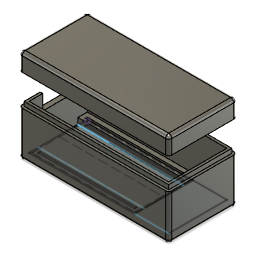
ReceiverCase (Autodesk Fusion 360 design; units mm, degrees)
Autodesk Fusion 360 part; units mm, degrees
note: some values were not read from the file. Set by a fixed rule: which face or edge a step refers to.
sketch "Sketch1" plane through (0, 0, 0) normal (0, 1, 0) x (1, 0, 0) in component "Case Bottom"
  line L0 (0, 0) -> (33.02, 0) construction
  line L1 (33.02, 0) -> (33.02, -17.78) construction
  line L2 (33.02, -17.78) -> (0, -17.78) construction
  line L3 (0, -17.78) -> (0, 0) construction
  line L4 (0, 0) -> (33.02, 0) construction
  line L5 (33.02, -2.54) -> (0, -2.54) construction
  line L6 (0, -2.54) -> (0, 0) construction
  line L7 (0, -17.78) -> (33.02, -17.78) construction
  line L8 (33.02, -17.78) -> (33.02, -15.24) construction
  line L9 (33.02, -15.24) -> (0, -15.24) construction
  line L10 (0, -15.24) -> (0, -17.78) construction
  line L11 (0, -8.89) -> (33.02, -8.89) construction
  line L12 (0.945, -0.945) -> (32.075, -0.945)
  line L13 (32.075, -0.945) -> (32.075, -1.595)
  line L14 (32.075, -1.595) -> (0.945, -1.595)
  line L15 (0.945, -1.595) -> (0.945, -0.945)
  line L16 (32.075, -16.835) -> (32.075, -16.185)
  line L17 (0.945, -16.185) -> (0.945, -16.835)
  line L18 (32.075, -16.185) -> (0.945, -16.185)
  line L19 (0.945, -16.835) -> (32.075, -16.835)
  line L20 (-0.5, -18.28) -> (-0.5, 0.5)
  line L21 (-0.5, 0.5) -> (33.52, 0.5)
  line L22 (33.52, 0.5) -> (33.52, -18.28)
  line L23 (33.52, -18.28) -> (-0.5, -18.28)
  line L24 (33.52, 0.5) -> (44.52, 0.5)
  line L25 (44.52, 0.5) -> (44.52, -18.28)
  line L26 (44.52, -18.28) -> (33.52, -18.28)
  line L27 (33.52, -18.28) -> (33.52, 0.5)
  line L28 (-0.5, -2.54) -> (33.52, -2.54)
  line L29 (33.52, -15.24) -> (-0.5, -15.24)
  dimension "d1" = 33.02
  dimension "d2" = 17.78
  dimension "d3" = 2.54
  dimension "d4" = 2.54
  dimension "d15" = 0.945
  dimension "d16" = 0.945
  dimension "d17" = 0.65
  dimension "d18" = 0.945
  dimension "d19" = -0.5
  dimension "d21" = 11
  constraint horizontal L0
  constraint vertical L1
  constraint horizontal L2
  constraint vertical L3
  constraint coincident L0.start L3.end
  constraint horizontal L4
  constraint horizontal L5
  constraint vertical L6
  constraint horizontal L7
  constraint vertical L8
  constraint coincident L1 L8.end
  constraint midpoint L3 L11.start
  constraint midpoint L1 L11.end
  constraint coincident L1 L5.start
  constraint horizontal L12
  constraint vertical L13
  constraint horizontal L14
  constraint vertical L15
  constraint symmetric L11 L12.start L17.end
  constraint symmetric L11 L12.end L16.start
  constraint symmetric L11 L13.end L16.end
  constraint symmetric L11 L14.end L17.start
  constraint horizontal L24
  constraint vertical L25
  constraint horizontal L26
  constraint vertical L27
  constraint coincident L20 L28.start
  constraint coincident L27 L28.end
  constraint perpendicular L27 L28
  constraint coincident L27 L29.start
  constraint coincident L20 L29.end
  constraint perpendicular L20 L29
  measures "d1" distance of L0.start L0.end
  measures "d2" distance of L0.start L2.end
  measures "d3" distance of L0.start L5.end
  measures "d4" distance of L2.end L9.end
  measures "d15" distance of L1 L13
  measures "d16" distance of L6 L15
  measures "d17" distance of L12 L14
  measures "d18" distance of L4 L12
  measures "d21" distance of L21.end L24.end
extrude "Extrude1" add sketch "Sketch1" along normal blind 17 contours L12 L13 L14 L15 | L16 L17 L18 L19 | L20 L22 L23 L27 L29 | L20 L22 L27 L28 L29 | L22 L24 L25 L26 L27 | L20 L21 L22 L27 L28 makes body 1 in component "Case Bottom"
shell "Shell1" thickness 1.6 outward yes removed faces 0 bodies 1 in component "Case Bottom"
ref_plane "WorkPlane2" through (22.01, 13, 8.89) normal (0, 1, 0) x (1, 0, 0) in component "Case Bottom"
split "Split2" by plane through (22.01, 13, 8.89) normal (0, 1, 0) bodies 1 makes body 2 at (13.9733, 18.6, 5.2267) in component "Case Bottom"
extrude "Extrude3" add sketch "Sketch1" along normal blind 2 contours L20 L22 L23 L27 L29 | L20 L21 L22 L27 L28 bodies 1 in component "Case Bottom"
sketch "Sketch2" plane through (-2.1, 0, 0) normal (-1, 0, 0) x (0, 0, 1) in component "Case Bottom"
  line L0 (19.88, 13) -> (-2.1, 13)
  line L1 (-2.1, 13) -> (-2.1, -1.6)
  line L2 (-2.1, -1.6) -> (19.88, -1.6)
  line L3 (19.88, -1.6) -> (19.88, 13)
  line L4 (18.28, 13) -> (-0.5, 13)
  line L5 (-0.5, 13) -> (-0.5, 0)
  line L6 (-0.5, 0) -> (18.28, 0)
  line L7 (18.28, 0) -> (18.28, 13)
  line L8 (8.89, 13) -> (8.89, 0) construction
  line L9 (3.89, 13) -> (13.89, 13)
  line L10 (13.89, 13) -> (13.89, 9.5)
  line L11 (13.89, 9.5) -> (3.89, 9.5)
  line L12 (3.89, 9.5) -> (3.89, 13)
  dimension "d30" = 9.5
  dimension "d31" = 5
  dimension "d32" = 5
  constraint midpoint L4 L8.start
  constraint midpoint L6 L8.end
  constraint horizontal L9
  constraint vertical L10
  constraint horizontal L11
  constraint vertical L12
  constraint coincident L4 L9.start
  measures "d30" distance of L6 L11
  measures "d31" distance of L8 L12
  measures "d32" distance of L8 L10
extrude "Extrude4" cut sketch "Sketch2" against normal up to surface (1.6 mm away) contours L0 L4 L9 L10 L11 L12 bodies 1 in component "Case Bottom"
fillet "Fillet1" radius 1 2 edges at (46.12, 5.7, 19.88) (46.12, 5.7, -2.1) on bodies 1 in component "Case Bottom"
fillet "Fillet2" radius 1 2 edges at (-2.1, 5.7, -2.1) (-2.1, 5.7, 19.88) on bodies 1 in component "Case Bottom"
ref_plane "WorkPlane3" through (22.01, 11.4, 8.89) normal (0, 1, 0) x (0, 0, 1) in component "Case Bottom"
split_face "SplitFace1" 4 faces at (25.8467, 9.3333, -0.5) (-0.5, 4.5, 10.5567) (25.8467, 9.3333, 18.28) (44.52, 4.3333, 5.76) by plane through (22.01, 11.4, 8.89) normal (0, 1, 0) on bodies 1 in component "Case Bottom"
move_face "OffsetFaces1" offset -0.8 5 faces at (14.5067, 11.9333, -0.5) (-0.5, 11.9333, 2.4267) (-0.5, 11.9333, 16.8167) (29.5133, 11.9333, 18.28) (44.52, 12.4667, 5.76) on bodies 1 in component "Case Bottom"
sketch "Sketch4" plane through (44.52, 0, 0) normal (-1, 0, 0) x (0, 0, 1) in component "Case Bottom"
  line L0 (18.28, 11.4) -> (-0.5, 11.4)
  line L1 (-0.5, 11.4) -> (-0.5, 0)
  line L2 (-0.5, 0) -> (18.28, 0)
  line L3 (18.28, 0) -> (18.28, 11.4)
  line L4 (4.755, 10) -> (13.025, 10)
  line L5 (13.025, 10) -> (13.025, 9.35)
  line L6 (13.025, 9.35) -> (4.755, 9.35)
  line L7 (4.755, 9.35) -> (4.755, 10)
  line L8 (8.89, 13) -> (8.89, 0) construction
  line L9 (-0.5, 0) -> (18.28, 0)
  line L10 (14.025, 8.35) -> (3.755, 8.35)
  line L11 (3.755, 8.35) -> (3.755, 11)
  line L12 (3.755, 11) -> (14.025, 11)
  line L13 (14.025, 11) -> (14.025, 8.35)
  dimension "d43" = 8.27
  dimension "d44" = 0.65
  dimension "d45" = 4.135
  dimension "d46" = 9.35
  dimension "d47" = -1
  constraint horizontal L4
  constraint vertical L5
  constraint horizontal L6
  constraint vertical L7
  measures "d43" distance of L4.start L4.end
  measures "d44" distance of L4.start L6.end
  measures "d45" distance of L7 L8
  measures "d46" distance of L6 L9
extrude "Extrude5" add sketch "Sketch4" along normal blind 1.6 contours L10 L11 L12 L13 bodies 1 in component "Case Bottom"
fillet "Fillet3" radius 1 4 edges at (-2.1, 15.8, 19.88) (-2.1, 15.8, -2.1) (46.12, 15.8, 19.88) (46.12, 15.8, -2.1) on bodies 2 in component "Case Bottom"
ref_plane "WorkPlane4" through (22.01, 14.6, 8.89) normal (0, -1, 0) x (0, 0, -1) in component "Case Bottom"
split_face "SplitFace2" 4 faces at (29.5133, 15.6667, 18.28) (-0.5, 14.3333, 12.02) (14.5067, 15.6667, -0.5) (44.52, 14.3333, 5.76) by plane through (22.01, 14.6, 8.89) normal (0, -1, 0) on bodies 2 in component "Case Bottom"
move_face "OffsetFaces2" offset -0.8 4 faces at (14.5067, 13.5333, -0.5) (44.52, 14.0667, 5.76) (29.5133, 13.5333, 18.28) (-0.5, 13.5333, 12.02) on bodies 2 in component "Case Bottom"
extrude "Extrude6" add 1 faces at (14.5067, 11.4, 18.8133) along direction (0, 1, 0) blind 3 on bodies 1 bodies 1 in component "Case Bottom"
move_face "OffsetFaces3" offset -0.1 4 faces at (-1.3, 14.0667, 12.2867) (14.24, 14.0667, 19.08) (29.78, 14.0667, -1.3) (45.32, 13.5333, 5.4933) on bodies 2 in component "Case Bottom"
fillet "Fillet4" radius 1 8 edges at (-1.8071, 18.6, 19.5871) (22.01, 18.6, 19.88) (45.8271, 18.6, 19.5871) (46.12, 18.6, 8.89) (45.8271, 18.6, -1.8071) (22.01, 18.6, -2.1) (-1.8071, 18.6, -1.8071) (-2.1, 18.6, 8.89) on bodies 2 in component "Case Bottom"
fillet "Fillet5" radius 1 8 edges at (-1.8071, -1.6, -1.8071) (22.01, -1.6, -2.1) (45.8271, -1.6, -1.8071) (46.12, -1.6, 8.89) (45.8271, -1.6, 19.5871) (22.01, -1.6, 19.88) (-1.8071, -1.6, 19.5871) (-2.1, -1.6, 8.89) on bodies 1 in component "Case Bottom"
extrude "Extrude7" add 1 faces at (43.9867, 8.35, 10.6017) along direction (0, -1, 0) blind 2 on bodies 1 bodies 1 in component "Case Bottom"
chamfer "Chamfer1" distance 1.5 distance2 2 1 edges at (42.92, 6.35, 8.89) measured on face at (43.9867, 6.35, 10.6017) on bodies 1 in component "Case Bottom"
copy_body "Body->Comp1" bodies 2 removing the originals makes body 3 in component "Case Top"
component "Case Bottom" placed x (1, 0, 0) y (0, 1, 0) z (0, 0, 1) at (0, 0, 0)
component "Case Top" placed x (1, 0, 0) y (0, 1, 0) z (0, 0, 1) at (0, 0, 0) in component "Case Bottom"
equation "d1 = ( 13 * 2.54 ) * 1 mm"
equation "d2 = ( 7 * 2.54 ) * 1 mm"
equation "d43 = 0.65 mm + ( 3 * 2.54 ) * 1 mm"
equation "d45 = ( ( 0.65 + 3 * 2.54 ) / 2 ) * 1 mm"
equation "d46 = 10 mm - 0.65 mm"
